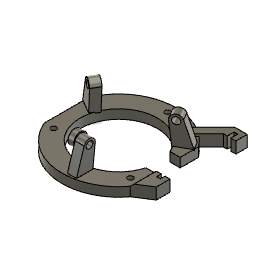
aball_v15 (Autodesk Fusion 360 design; units mm, degrees)
Autodesk Fusion 360 part; units mm, degrees
(part 1 of 2)
sphere "SpherePrimitive1" add diameter 38.1 placed x (1, 0, 0) y (0, 0, -1) z (0, 1, 0) at (0, 0, 0) makes body 1
ref_plane "WorkPlane1" through (0, -19.05, 0) normal (0, 1, 0) x (0, 0, 1)
mesh "Mesh1" [no effect]
ref_plane "WorkPlane2" through (0, -17.55, 0) normal (0, 1, 0) x (0, 0, 1)
sketch "bearing_38" plane through (0, 0, 0) normal (1, 0, 0) x (0, 0, -1)
  circle A0 centre (0, 0) radius 22.05 construction
  circle A1 centre (-18.1301, -12.55) radius 3
  circle A2 centre (-18.1301, -12.55) radius 1.5
  line L0 (-30, 0) -> (28, 0) construction
  line L1 (-30, -19.05) -> (30, -19.05) construction
  dimension "d13" = 44.1
  dimension "d14" = 6
  dimension "d15" = 3
  dimension "d16" = 19.05
  dimension "d17" = 6.5
  constraint coincident A0.centre origin
  constraint coincident A0 A1.centre
  constraint concentric A1 A2
  constraint horizontal L0
  constraint horizontal L1
  measures "d13" diameter of A0
  measures "d14" diameter of A1
  measures "d15" diameter of A2
  measures "d16" distance of L0 L1
  measures "d17" distance of A1.centre L1
sketch "bearing_holder_38" plane through (0, 0, 0) normal (1, 0, 0) x (0, 0, -1)
  circle A0 centre (-18.1301, -12.55) radius 2.5
  line L0 (-24.0474, -23.0415) -> (-20.5151, -11.8006)
  line L1 (-15.6305, -12.5064) -> (-16.7406, -23.0415)
  line L2 (-16.7406, -23.0415) -> (-24.0474, -23.0415)
  line L3 (0, -14.55) -> (0, -11.55)
  circle A1 centre (-18.1301, -12.55) radius 1.5
  point P0 (0, -13.05)
  point P1 (-18.1301, -12.55)
  dimension "d18" = 5
  constraint coincident A0 L0.end
  constraint tangent A0 L0
  constraint coincident A0 L1.start
  constraint horizontal L2
  constraint coincident P1 A0.centre
  measures "d18" diameter of A0
extrude "Extrude1" add sketch "bearing_38" along normal mid plane 2.5 separate body makes body 2
sketch "a9800_dimensino" plane through (0, 0, 0) normal (0, 1, 0) x (1, 0, 0)
  circle A0 centre (0, 0) radius 15.8
  line L0 (9.75, -10.75) -> (-9.75, -10.75)
  line L1 (-9.75, -10.75) -> (-9.75, 10.75)
  line L2 (-9.75, 10.75) -> (9.75, 10.75)
  line L3 (9.75, 10.75) -> (9.75, -10.75)
  line L4 (9.75, -10.75) -> (-9.75, 10.75) construction
  line L5 (-9.75, -10.75) -> (9.75, 10.75) construction
  line L6 (7.5, -8) -> (-7.5, -8)
  line L7 (-7.5, -8) -> (-7.5, 8)
  line L8 (-7.5, 8) -> (7.5, 8)
  line L9 (7.5, 8) -> (7.5, -8)
  line L10 (7.5, -8) -> (-7.5, 8) construction
  line L11 (-7.5, -8) -> (7.5, 8) construction
  circle A1 centre (0, 13.05) radius 1.25
  line L12 (-1.5901, 14.3) -> (1.6928, 14.3) construction
  line L13 (-2.2181, 15.8) -> (-2, 15.8)
  line L14 (-2, 15.8) -> (2, 15.8) construction
  circle A2 centre (0, -13.05) radius 1.25
  line L15 (-3.1209, -14.3) -> (2.5, -14.3) construction
  line L16 (-3, -15.8) -> (2.5, -15.8) construction
  line L17 (0, 40) -> (0, -43.8332) construction
  dimension "d32" = 31.6
  dimension "d33" = 21.5
  dimension "d34" = 19.5
  dimension "d35" = 15
  dimension "d36" = 16
  dimension "d37" = 2.5
  dimension "d38" = 1.5
  dimension "d39" = 2.5
  dimension "d40" = 1.5
  constraint coincident A0.centre origin
  constraint perpendicular L0 L1
  constraint parallel L0 L2
  constraint parallel L1 L3
  constraint horizontal L0
  constraint coincident L4 A0.centre
  constraint coincident L5 A0.centre
  constraint perpendicular L6 L7
  constraint parallel L6 L8
  constraint parallel L7 L9
  constraint horizontal L6
  constraint coincident L10 A0.centre
  constraint coincident L11 A0.centre
  constraint horizontal L12
  constraint parallel L12 L13
  constraint parallel L12 L14
  constraint tangent A0 L14
  constraint tangent A1 L12
  constraint horizontal L15
  constraint horizontal L16
  constraint tangent A0 L16
  constraint vertical L17
  constraint coincident A2.centre L17
  constraint tangent A2 L15
  measures "d32" diameter of A0
  measures "d33" distance of L0.end L1.end
  measures "d34" distance of L1.end L2.end
  measures "d35" distance of L7.end L8.end
  measures "d36" distance of L6.end L7.end
  measures "d37" diameter of A1
  measures "d38" distance of L12 L14
  measures "d39" diameter of A2
  measures "d40" distance of L15 L16
extrude "Extrude4" add sketch "a9800_dimensino" along normal blind 1.7 separate body contours A0 | L0 L1 L2 L3 | L6 L7 L8 L9 makes body 3
extrude "Extrude5" add sketch "a9800_dimensino" along normal blind 5 separate body contours L0 L1 L2 L3 | L6 L7 L8 L9 makes body 4
extrude "Extrude6" add sketch "a9800_dimensino" against normal blind 3 separate body contours L6 L7 L8 L9 makes body 5
combine "Combine3" operation add target body 3 tool bodies 4 5
copy_body "CopyPasteBodies3" bodies 3 makes body 6
move_body "Move4" bodies 6 to x (1, 0, 0) y (0, 1, 0) z (0, 0, 1) at (0, -30, 0)
move_body "Move5" bodies 6 to x (1, 0, 0) y (0, 1, 0) z (0, 0, 1) at (0, 3, 0)
move_body "Move6" bodies 6 to x (1, 0, 0) y (0, 1, 0) z (0, 0, 1) at (0, 2, 0)
move_body "Move7" bodies 6 to x (1, 0, 0) y (0, 1, 0) z (0, 0, 1) at (0, 0.15, 0)
move_body "Move8" bodies 6 to x (1, 0, 0) y (0, 1, 0) z (0, 0, 1) at (0, 0.5, 0)
move_face "MoveFace1" by (0, 0.02, 0) 1 faces at (-9.75, -20.45, 3.5833) on bodies 6
move_body "Move9" bodies 6 to x (1, 0, 0) y (0, 1, 0) z (0, 0, 1) at (0, 0.2, 0)
move_body "Move10" bodies 6 to x (1, 0, 0) y (0, 1, 0) z (0, 0, 1) at (0, -2.3, 0)
move_body "Move11" bodies 6 to x (1, 0, 0) y (0, 1, 0) z (0, 0, 1) at (0, 0.1, 0)
move_body "Move12" bodies 6 to x (0.34202, 0.939693, 0) y (-0.939693, 0.34202, 0) z (0, 0, 1) at (0, 0, 0)
ref_plane "WorkPlane5" through (0, -28, 0) normal (0, 1, 0) x (0, 0, 1)
ref_plane "WorkPlane6" through (0, -11, 0) normal (0, 1, 0) x (0, 0, 1)
ref_plane "WorkPlane7" through (0, -26.5, 0) normal (0, 1, 0) x (0, 0, 1)
move_body "Move13" bodies 6 to x (0, 0, -1) y (0, 1, 0) z (1, 0, 0) at (0, 0, 0)
mesh "Mesh2" [no effect]
sketch "Kyria_footprint" plane through (46, -28, 42) normal (0, 1, 0) x (1, 0, 0)
  line L0 (-210.8879, -20.4424) -> (-220.8051, -30.3595)
  circle A0 centre (-87.084, 9.634) radius 1.1
  arc A1 (-165.3859, -1.5948) -> (-210.8879, -20.4424) centre (-165.3859, -65.9444) ccw
  arc A2 (-128.8109, 1.9052) -> (-132.3109, -1.5948) centre (-132.3109, 1.9052) cw
  line L1 (-83.425, 74.1919) -> (-83.425, 9.475)
  arc A3 (-205.7208, 93.1275) -> (-85.2151, 77.2458) centre (-165.3859, -65.9444) cw
  circle A4 centre (-231.9682, 80.7528) radius 1.1
  circle A5 centre (-86.7356, 74.2991) radius 1.1
  circle A6 centre (-243.225, 19.2739) radius 1.1
  circle A7 centre (-256.3598, 5.4201) radius 1.1
  arc A8 (-85.2151, 77.2458) -> (-83.425, 74.1919) centre (-86.925, 74.1919) cw
  circle A9 centre (-223.2799, -27.6598) radius 1.1
  arc A10 (-245.225, 52.0721) -> (-246.225, 53.0721) centre (-245.225, 53.0721) cw
  arc A11 (-259.0595, 2.9452) -> (-259.0595, 7.8949) centre (-256.5847, 5.4201) cw
  line L2 (-228.225, 77.6065) -> (-207.475, 77.6065)
  arc A12 (-220.8051, -30.3595) -> (-225.7548, -30.3595) centre (-223.2799, -27.8847) cw
  arc A13 (-239.225, 51.0721) -> (-240.225, 52.0721) centre (-240.225, 51.0721) ccw
  line L3 (-225.7548, -30.3595) -> (-259.0595, 2.9452)
  line L4 (-240.225, 52.0721) -> (-245.225, 52.0721)
  arc A14 (-206.475, 92.1582) -> (-205.7208, 93.1275) centre (-205.475, 92.1582) cw
  arc A15 (-249.1424, 17.8121) -> (-239.5985, 26.3746) centre (-165.3859, -65.9444) cw
  line L5 (-246.225, 53.0721) -> (-246.225, 74.8141)
  arc A16 (-244.4104, 77.8815) -> (-230.6225, 84.6377) centre (-165.3859, -65.9444) cw
  arc A17 (-229.225, 78.6065) -> (-228.225, 77.6065) centre (-228.225, 78.6065) ccw
  arc A18 (-125.3109, 5.975) -> (-128.8109, 2.475) centre (-125.3109, 2.475) ccw
  arc A19 (-230.6225, 84.6377) -> (-229.225, 83.7201) centre (-230.225, 83.7201) cw
  arc A20 (-207.475, 77.6065) -> (-206.475, 78.6065) centre (-207.475, 78.6065) ccw
  line L6 (-259.0595, 7.8949) -> (-249.1424, 17.8121)
  arc A21 (-246.225, 74.8141) -> (-244.4104, 77.8815) centre (-242.725, 74.8141) cw
  line L7 (-229.225, 83.7201) -> (-229.225, 78.6065)
  line L8 (-128.8109, 2.475) -> (-128.8109, 1.9052)
  line L9 (-132.3109, -1.5948) -> (-165.3859, -1.5948)
  line L10 (-86.925, 5.975) -> (-125.3109, 5.975)
  arc A22 (-83.425, 9.475) -> (-86.925, 5.975) centre (-86.925, 9.475) cw
  arc A23 (-239.5985, 26.3746) -> (-239.225, 27.154) centre (-240.225, 27.154) ccw
  line L11 (-239.225, 27.154) -> (-239.225, 51.0721)
  line L12 (-206.475, 78.6065) -> (-206.475, 92.1582)
  circle A24 centre (-243.225, 55.0721) radius 1.1
  circle A25 centre (-203.5672, 90.5701) radius 1.1
copy_body "CopyPasteBodies6" bodies 2 makes body 7
move_body "Move16" bodies 7 to x (-0.5, 0, -0.866025) y (0, 1, 0) z (0.866025, 0, -0.5) at (0, 0, 0)
copy_body "CopyPasteBodies7" bodies 2 makes body 8
move_body "Move22" bodies 6 to x (1, 0, 0) y (0, 0.34202, -0.939693) z (0, 0.939693, 0.34202) at (0, 0, 0)
move_body "Move17" bodies 8 to x (-0.5, 0, 0.866025) y (0, 1, 0) z (-0.866025, 0, -0.5) at (0, 0, 0)
move_body "Move23" bodies 6 to x (0, 0, -1) y (0, 1, 0) z (1, 0, 0) at (0, 0, 0)
sketch "holder" plane through (0, -26.5, 0) normal (0, 1, 0) x (1, 0, 0)
  circle A0 centre (0, 0) radius 25
  circle A1 centre (0, 0) radius 17
  line L0 (0, 0) -> (25, 0) construction
  line L1 (0, 0) -> (25, 0) construction
  line L2 (20, 18) -> (20, -15)
  circle A2 centre (-18.8875, -9.75) radius 1.2
  circle A3 centre (0, 21.5) radius 1.2
  circle A4 centre (16.8875, -11.75) radius 1.2
  line L3 (-23, 13) -> (-23, -12)
  dimension "d162" = 50
  dimension "d163" = 34
  dimension "d242" = 2.4
  dimension "d243" = 2.4
  dimension "d244" = 2.4
  constraint coincident A0.centre A1.centre
  constraint concentric A0 A1
  constraint horizontal L0
  constraint horizontal L1
  constraint vertical L2
  constraint vertical L3
  measures "d162" diameter of A0
  measures "d163" diameter of A1
  measures "d242" diameter of A2
  measures "d243" diameter of A3
  measures "d244" diameter of A4
extrude "Extrude27" add sketch "holder" along normal blind 4 separate body contours A0 L2 L3 makes body 9
extrude "Extrude28" add sketch "bearing_holder_38" along normal blind 4 from surface at 1.25 separate body contours A0 L1 | A0 L0 L1 L2 picked at (-15.9906, -12.7979) makes body 10
pattern_circular "C-Pattern1" count 3 over 360 about axis through (0, 1.75, 0) along (0, 1, 0) of bodies 10 makes body 11 at (14.5414, -20.0098, -14.4576) makes body 12 at (-19.7914, -20.0098, -5.3644)
sketch "micro_holder" plane through (0, -26.5, 0) normal (0, 1, 0) x (1, 0, 0)
  line L0 (23.2, -6.5) -> (24.8, -6.5)
  line L1 (20, -10.5) -> (20, -6.5)
  line L2 (23.2, -6.5) -> (23.2, -4.5)
  line L3 (23.2, -4.5) -> (20, -4.5)
  line L4 (20, -4.5) -> (20, -6.5)
  line L5 (24.8, -4.5) -> (27, -4.5)
  line L6 (24.8, -6.5) -> (24.8, -4.5)
  line L7 (24.8, 27.5) -> (23.2, 27.5)
  line L8 (21.5, 27.5) -> (21.5, 29.5)
  line L9 (21.5, 29.5) -> (27, 29.5)
  line L10 (27, 24.5) -> (24.8, 24.5)
  line L11 (24.8, 24.5) -> (24.8, 27.5)
  line L12 (23.2, 27.5) -> (23.2, 24.5)
  line L13 (23.2, 24.5) -> (21.5, 24.5)
  line L14 (21.5, 24.5) -> (21.5, 27.5)
  line L15 (21.5, 29.5) -> (9.7205, 17.7205)
  line L16 (21.5, 29.5) -> (34.4035, 29.5) construction
  line L17 (21.5, 24.5) -> (12.8239, 15.8239)
  line L18 (21.5, 24.5) -> (30.0147, 24.5) construction
  line L19 (9.7205, 17.7205) -> (12.8239, 15.8239)
  line L20 (27, -10.5) -> (20, -15)
  line L21 (20, -15) -> (20, -10.5)
  line L22 (27, 24.5) -> (27, 29.5)
  line L23 (27, -4.5) -> (27, -10.5)
  dimension "d200" = 4
  dimension "d201" = 135
  dimension "d202" = 135
  dimension "d383" = 1.6
  constraint horizontal L0
  constraint vertical L1
  constraint vertical L2
  constraint horizontal L3
  constraint vertical L4
  constraint horizontal L5
  constraint vertical L6
  constraint horizontal L7
  constraint vertical L8
  constraint horizontal L9
  constraint horizontal L10
  constraint vertical L11
  constraint vertical L12
  constraint horizontal L13
  constraint vertical L14
  constraint coincident L7 L8.start
  constraint horizontal L16
  constraint horizontal L18
  constraint collinear L6 L11
  constraint perpendicular L16 L22
  constraint collinear L2 L12
  measures "d200" distance of L1.end L1.start
  measures "d201" angle of L15 L16
  measures "d202" angle of L17 L18
  measures "d383" distance of L2 L5.start
sketch "case_body_guides" plane through (0, -28, 0) normal (0, 1, 0) x (1, 0, 0)
  line L0 (0, 70) -> (0, -60) construction
  line L1 (34, 26.9443) -> (34, -18.401)
  line L2 (11.4009, -41) -> (-25, -41)
  line L3 (-29, -37) -> (-29, 26.9855)
  arc A0 (30.9987, 30.8176) -> (-25.993, 30.8603) centre (2.4198, -80.0119) ccw
  arc A1 (-25.993, 30.8603) -> (-29, 26.9855) centre (-25, 26.9855) ccw
  arc A2 (-29, -37) -> (-25, -41) centre (-25, -37) ccw
  arc A3 (34, 26.9443) -> (30.9987, 30.8176) centre (30, 26.9443) ccw
  line L4 (-23, -31) -> (-23, 22.3021)
  arc A4 (28.16, 25.4237) -> (-19.8196, 26.2173) centre (2.4198, -80.0119) ccw
  line L5 (18.1274, 27.3776) -> (21.5156, 31.1472)
  line L6 (29.1545, 31.2768) -> (29.1545, 28.4999)
  line L7 (29.1545, 28.4999) -> (28.1728, 28.4999)
  line L8 (28.16, 25.4237) -> (28.1728, 28.4999)
  line L9 (32.8284, -21.2294) -> (14.2294, -39.8284)
  line L10 (26.8132, -18.7593) -> (11.7441, -33.8284)
  arc A5 (11.4009, -41) -> (14.2294, -39.8284) centre (11.4009, -37) ccw
  arc A6 (32.8284, -21.2294) -> (34, -18.401) centre (30, -18.401) ccw
  line L11 (-19, -35) -> (8.9157, -35)
  line L12 (27.9847, -15.9479) -> (28.16, 25.4237)
  circle A7 centre (-25, -37) radius 1.2
  arc A8 (-23, -31) -> (-19, -35) centre (-19, -31) ccw
  arc A9 (8.9157, -35) -> (11.7441, -33.8284) centre (8.9157, -31) ccw
  arc A10 (26.8132, -18.7593) -> (27.9847, -15.9479) centre (23.9848, -15.9309) ccw
  arc A11 (-19.8196, 26.2173) -> (-23, 22.3021) centre (-19, 22.3021) ccw
  circle A12 centre (-25, -37) radius 1.75
  circle A13 centre (-25, 26.9855) radius 1.2
  circle A14 centre (-25, 26.9855) radius 1.75
  circle A15 centre (17, 31) radius 1.2
  circle A16 centre (17, 31) radius 1.75
  circle A17 centre (31, 26) radius 1.2
  circle A18 centre (31, 26) radius 1.75
  circle A19 centre (11, -38) radius 1.2
  circle A20 centre (11, -38) radius 1.75
  circle A21 centre (31, -18) radius 1.2
  circle A22 centre (31, -18) radius 1.75
  line L13 (21.5156, 31.1472) -> (21.5156, 32.8388)
  circle A23 centre (31, 4) radius 1.2
  circle A24 centre (31, 4) radius 1.75
  line L14 (28.0545, 0.5306) -> (34, 0.5306)
  line L15 (28.0414, -2.5651) -> (34, -2.5651)
  point P0 (34, 30)
  point P1 (34, -41)
  dimension "d213" = 71
  dimension "d214" = 4
  dimension "d217" = 6
  dimension "d218" = 4
  dimension "d219" = 4
  dimension "d220" = 2.4
  dimension "d221" = 4
  dimension "d222" = 3.5
  dimension "d223" = 2.4
  dimension "d224" = 3.5
  dimension "d225" = 2.4
  dimension "d226" = 3.5
  dimension "d227" = 2.4
  dimension "d228" = 3.5
  dimension "d229" = 2.4
  dimension "d230" = 3.5
  dimension "d231" = 2.4
  dimension "d232" = 3.5
  dimension "d320" = 2.4
  dimension "d321" = 3.5
  constraint vertical L0
  constraint vertical L1
  constraint horizontal L2
  constraint vertical L3
  constraint tangent A0 A1
  constraint tangent L3 A1
  constraint tangent L3 A2
  constraint tangent L2 A2
  constraint equal A1 A2
  constraint coincident P1 L2
  constraint coincident P1 L1
  constraint coincident P0 L1
  constraint coincident P0 A0
  constraint tangent L1 A3
  constraint tangent A0 A3
  constraint equal A1 A3
  constraint coincident A4 L5.start
  constraint coincident A0 L6.start
  constraint perpendicular L6 L7
  constraint parallel L9 L10
  constraint parallel L3 L4
  constraint concentric A0 A4
  constraint tangent L9 A5
  constraint tangent L2 A5
  constraint tangent L1 A6
  constraint tangent L9 A6
  constraint concentric A2 A7
  constraint tangent L4 A8
  constraint tangent L11 A8
  constraint tangent L11 A9
  constraint tangent L10 A9
  constraint equal A8 A9
  constraint tangent L10 A10
  constraint tangent L12 A10
  constraint equal A8 A10
  constraint tangent A4 A11
  constraint tangent L4 A11
  constraint equal A8 A11
  constraint concentric A7 A12
  constraint concentric A1 A13
  constraint concentric A1 A14
  constraint concentric A15 A16
  constraint concentric A17 A18
  constraint concentric A19 A20
  constraint concentric A21 A22
  constraint coincident A0 L13.end
  constraint vertical L13
  constraint concentric A23 A24
  constraint coincident L12 L14.start
  constraint coincident L1 L14.end
  constraint perpendicular L1 L14
  constraint coincident L12 L15.start
  constraint coincident L1 L15.end
  constraint perpendicular L1 L15
  measures "d213" distance of P0 P1
  measures "d214" radius of A1
  measures "d217" distance of L9 L10
  measures "d218" radius of A5
  measures "d219" radius of A6
  measures "d220" diameter of A7
  measures "d221" radius of A8
  measures "d222" diameter of A12
  measures "d223" diameter of A13
  measures "d224" diameter of A14
  measures "d225" diameter of A15
  measures "d226" diameter of A16
  measures "d227" diameter of A17
  measures "d228" diameter of A18
  measures "d229" diameter of A19
  measures "d230" diameter of A20
  measures "d231" diameter of A21
  measures "d232" diameter of A22
  measures "d320" diameter of A23
  measures "d321" diameter of A24
sketch "BOTTOM" plane through (0, -28, 0) normal (0, 1, 0) x (1, 0, 0)
  arc A0 (30.9987, 30.8176) -> (-25.993, 30.8603) centre (2.4198, -80.0119) ccw
  arc A1 (-25.993, 30.8603) -> (-29, 26.9855) centre (-25, 26.9855) ccw
  line L0 (-29, -37) -> (-29, 26.9855)
  arc A2 (34, 26.9443) -> (30.9987, 30.8176) centre (30, 26.9443) ccw
  line L1 (34, 26.9443) -> (34, -18.401)
  arc A3 (32.8284, -21.2294) -> (34, -18.401) centre (30, -18.401) ccw
  line L2 (32.8284, -21.2294) -> (14.2294, -39.8284)
  arc A4 (11.4009, -41) -> (14.2294, -39.8284) centre (11.4009, -37) ccw
  line L3 (11.4009, -41) -> (-25, -41)
  arc A5 (-29, -37) -> (-25, -41) centre (-25, -37) ccw
  circle A6 centre (-25, -37) radius 1.2
  circle A7 centre (11, -38) radius 1.2
  circle A8 centre (31, -18) radius 1.2
  circle A9 centre (31, 26) radius 1.2
  circle A10 centre (17, 31) radius 1.2
  circle A11 centre (-25, 26.9855) radius 1.2
  circle A12 centre (-18.8875, -9.75) radius 1.2
  circle A13 centre (16.8875, -11.75) radius 1.2
  circle A14 centre (0, 21.5) radius 1.2
  circle A15 centre (0, 13.0504) radius 1.2
  circle A16 centre (0, -13.05) radius 1.2
  arc A17 (-6.9032, 13.9049) -> (6.9032, 13.9049) centre (0, 18.0543) ccw
  arc A18 (6.9032, -13.9049) -> (-6.9032, -13.9049) centre (0, -18.0543) ccw
  arc A19 (-6.9032, 13.9049) -> (-6.9032, -13.9049) centre (0, 0) ccw
  arc A20 (6.9032, -13.9049) -> (6.9032, 13.9049) centre (0, 0) ccw
  circle A21 centre (31, 4) radius 1.2
  point P0 (-18.8875, -9.75)
  point P1 (34, 0.5306)
  dimension "d258" = 2.4
  dimension "d259" = 2.4
  constraint coincident A19.centre A20.centre
  constraint coincident A18.start A19
  constraint concentric A19 A20
  measures "d258" diameter of A15
  measures "d259" diameter of A16
extrude "Extrude29" add sketch "micro_holder" along normal blind 5 separate body makes body 13 at (17.5735, -24.8333, -25.5735) makes body 14 at (23.4, -26.5, 10.6667)
combine "Combine8" operation add target body 9 tool bodies 13 10 12 11 14
chamfer "Chamfer3" distance 1 angle 45 1 edges at (20, -21.5, 9.75) on bodies 9
chamfer "Chamfer4" distance 1 angle 45 1 edges at (11.2722, -21.5, -16.7722) on bodies 9
extrude "Extrude30" add sketch "BOTTOM" along normal blind 1.5 separate body makes body 15
extrude "Extrude31" add sketch "Kyria_footprint" along normal blind 17 separate body makes body 16
sketch "MIDDLEA" plane through (0, -26.5, 0) normal (0, 1, 0) x (1, 0, 0)
  line L0 (-29, -37) -> (-29, 26.9855)
  arc A0 (-25.993, 30.8603) -> (-29, 26.9855) centre (-25, 26.9855) ccw
  circle A1 centre (-25, 26.9855) radius 1.75
  arc A2 (-19.8196, 26.2173) -> (-23, 22.3021) centre (-19, 22.3021) ccw
  arc A3 (18.1274, 27.3776) -> (-19.8196, 26.2173) centre (2.4198, -80.0119) ccw
  line L1 (-23, -31) -> (-23, 22.3021)
  line L2 (18.1274, 27.3776) -> (21.5156, 31.1472)
  line L3 (29.1545, 31.2768) -> (29.1545, 28.4999)
  line L4 (29.1545, 28.4999) -> (28.1728, 28.4999)
  line L5 (28.16, 25.4237) -> (28.1728, 28.4999)
  circle A4 centre (31, 26) radius 1.75
  arc A5 (34, 26.9443) -> (30.9987, 30.8176) centre (30, 26.9443) ccw
  line L6 (27.9847, -15.9479) -> (28.16, 25.4237)
  line L7 (34, 26.9443) -> (34, -18.401)
  arc A6 (32.8284, -21.2294) -> (34, -18.401) centre (30, -18.401) ccw
  arc A7 (26.8132, -18.7593) -> (27.9847, -15.9479) centre (23.9848, -15.9309) ccw
  circle A8 centre (31, -18) radius 1.75
  line L8 (32.8284, -21.2294) -> (14.2294, -39.8284)
  line L9 (26.8132, -18.7593) -> (11.7441, -33.8284)
  arc A9 (11.4009, -41) -> (14.2294, -39.8284) centre (11.4009, -37) ccw
  arc A10 (8.9157, -35) -> (11.7441, -33.8284) centre (8.9157, -31) ccw
  circle A11 centre (11, -38) radius 1.75
  line L10 (11.4009, -41) -> (-25, -41)
  line L11 (-19, -35) -> (8.9157, -35)
  arc A12 (-23, -31) -> (-19, -35) centre (-19, -31) ccw
  arc A13 (-29, -37) -> (-25, -41) centre (-25, -37) ccw
  circle A14 centre (-25, -37) radius 1.75
  circle A15 centre (17, 31) radius 1.75
  line L12 (21.5156, 31.1472) -> (21.5156, 32.8388)
  arc A16 (30.9987, 30.8176) -> (29.1545, 31.2768) centre (2.4198, -80.0119) ccw
  arc A17 (21.5156, 32.8388) -> (-25.993, 30.8603) centre (2.4198, -80.0119) ccw
  circle A18 centre (31, 4) radius 1.75
  constraint concentric A16 A17
ref_plane "WorkPlane10" through (0, -11.5, 0) normal (0, 1, 0) x (0, 0, 1)
sketch "topA" plane through (0, -11.5, 0) normal (0, 1, 0) x (-1, 0, 0)
  circle A0 centre (-31, -26) radius 1.75
  circle A1 centre (25, 37) radius 1.75
  circle A2 centre (-17, -31) radius 1.75
  circle A3 centre (-31, 18) radius 1.75
  circle A4 centre (-11, 38) radius 1.75
  circle A5 centre (25, -26.9855) radius 1.75
  line L0 (-18.1274, -27.3776) -> (-21.5156, -31.1472)
  line L1 (-21.5156, -31.1472) -> (-23.0477, -31.1472)
  line L2 (-23.0477, -31.1472) -> (-23.0477, -32.5688)
  arc A6 (-23.0477, -32.5688) -> (25.993, -30.8603) centre (-2.4198, 80.0119) ccw
  arc A7 (25.993, -30.8603) -> (29, -26.9855) centre (25, -26.9855) ccw
  line L3 (29, -26.9855) -> (29, 37)
  arc A8 (29, 37) -> (25, 41) centre (25, 37) ccw
  line L4 (25, 41) -> (-11.4009, 41)
  arc A9 (-11.4009, 41) -> (-14.2294, 39.8284) centre (-11.4009, 37) ccw
  line L5 (-14.2294, 39.8284) -> (-32.8284, 21.2294)
  arc A10 (-32.8284, 21.2294) -> (-34, 18.401) centre (-30, 18.401) ccw
  line L6 (-34, 18.401) -> (-34, -26.9443)
  arc A11 (-34, -26.9443) -> (-30.9987, -30.8176) centre (-30, -26.9443) ccw
  arc A12 (-30.9987, -30.8176) -> (-29.1545, -31.2768) centre (-2.4198, 80.0119) ccw
  line L7 (-29.1545, -31.2768) -> (-29.1545, -28.4999)
  line L8 (-29.1545, -28.4999) -> (-28.1728, -28.4999)
  line L9 (-28.1728, -28.4999) -> (-28.16, -25.4237)
  line L10 (-28.16, -25.4237) -> (-27.9847, 15.9479)
  arc A13 (-26.8132, 18.7593) -> (-27.9847, 15.9479) centre (-23.9848, 15.9309) ccw
  line L11 (-26.8132, 18.7593) -> (-11.7441, 33.8284)
  arc A14 (-8.9157, 35) -> (-11.7441, 33.8284) centre (-8.9157, 31) ccw
  line L12 (-8.9157, 35) -> (19, 35)
  arc A15 (23, 31) -> (19, 35) centre (19, 31) ccw
  line L13 (23, 31) -> (23, -22.3021)
  arc A16 (19.8196, -26.2173) -> (23, -22.3021) centre (19, -22.3021) ccw
  arc A17 (-18.1274, -27.3776) -> (19.8196, -26.2173) centre (-2.4198, 80.0119) ccw
  line L14 (29, 37) -> (29, -26.9855)
  arc A18 (25.993, -30.8603) -> (29, -26.9855) centre (25, -26.9855) ccw
  arc A19 (-30.9987, -30.8176) -> (25.993, -30.8603) centre (-2.4198, 80.0119) ccw
  line L15 (-11.4009, 41) -> (25, 41)
  arc A20 (29, 37) -> (25, 41) centre (25, 37) ccw
  arc A21 (-11.4009, 41) -> (-14.2294, 39.8284) centre (-11.4009, 37) ccw
  line L16 (-32.8284, 21.2294) -> (-14.2294, 39.8284)
  arc A22 (-32.8284, 21.2294) -> (-34, 18.401) centre (-30, 18.401) ccw
  line L17 (-34, -26.9443) -> (-34, 18.401)
  circle A23 centre (-31, 18) radius 1.2
  circle A24 centre (-11, 38) radius 1.2
  arc A25 (-34, -26.9443) -> (-30.9987, -30.8176) centre (-30, -26.9443) ccw
  circle A26 centre (-31, -26) radius 1.2
  circle A27 centre (-17, -31) radius 1.2
  circle A28 centre (25, -26.9855) radius 1.2
  circle A29 centre (25, 37) radius 1.2
  line L18 (-22.5, -28) -> (-25, -28)
  line L19 (-25, -28) -> (-25, 7)
  line L20 (-25, 7) -> (-22.5, 7)
  line L21 (-22.5, 7) -> (-22.5, -28)
  circle A30 centre (0, 0) radius 23
  circle A31 centre (0, 0) radius 17.5
  line L22 (0, 0) -> (21.5407, 0) construction
  line L23 (0, 0) -> (21.5407, 0) construction
  line L24 (0, 0) -> (21.5407, 0) construction
  line L25 (0, 0) -> (21.5407, 0) construction
  line L26 (0, 0) -> (21.5407, 0) construction
  line L27 (0, 0) -> (21.5407, 0) construction
  circle A32 centre (-2.4311, 13.7873) radius 9.5
  circle A33 centre (-10.7246, -8.999) radius 9.5
  circle A34 centre (13.1557, -4.7883) radius 9.5
  line L28 (-23.0477, -31.1472) -> (-22.5, -28)
  line L29 (-25, -28) -> (-29.1, -28)
  line L30 (-29.1, -28) -> (-29.1545, -28.4999)
  line L31 (-21.5156, -31.1472) -> (-21.5156, -32.8388)
  point P0 (-31, 18)
  dimension "d268" = 35
  dimension "d300" = 46
  dimension "d301" = 19
  dimension "d302" = 19
  dimension "d303" = 19
  constraint horizontal L18
  constraint vertical L19
  constraint horizontal L20
  constraint vertical L21
  constraint coincident A30.centre A31.centre
  constraint concentric A30 A31
  constraint horizontal L22
  constraint horizontal L23
  constraint horizontal L24
  constraint horizontal L25
  constraint horizontal L26
  constraint horizontal L27
  constraint vertical L31
  constraint coincident A6 L31.end
  measures "d268" diameter of A31
  measures "d300" diameter of A30
  measures "d301" diameter of A32
  measures "d302" diameter of A33
  measures "d303" diameter of A34
ref_plane "WorkPlane11" through (0, -10, 0) normal (0, 1, 0) x (0, 0, 1)
ref_plane "WorkPlane12" through (0, -8.5, 0) normal (0, 1, 0) x (0, 0, 1)
sketch "topC" plane through (0, -8.5, 0) normal (0, 1, 0) x (1, 0, 0)
  circle A0 centre (0, 0) radius 19
  line L0 (22.9701, 27.7101) -> (24.4724, 27.7101)
  line L1 (24.4724, 27.7101) -> (24.4724, -6.6306)
  line L2 (24.4724, -6.6306) -> (22.9701, -6.6306)
  line L3 (22.9701, -6.6306) -> (22.9701, 27.7101)
  line L4 (12.6019, -21.7825) -> (26.0559, -25.2289)
  line L5 (34.0004, 26.9508) -> (34, -18.401)
  arc A1 (34.0004, 26.9508) -> (30.9492, 30.8241) centre (29.9824, 26.924) ccw
  circle A2 centre (31, 26) radius 1.2
  circle A3 centre (31, -18) radius 1.2
  arc A4 (32.8284, -21.2294) -> (34, -18.401) centre (30, -18.401) ccw
  line L6 (1.4117, 24.935) -> (13.6846, 32.4672)
  arc A5 (26.0559, -25.2289) -> (29.8, -24.2573) centre (27.0485, -21.354) ccw
  arc A6 (30.9492, 30.8241) -> (17.6483, 33.4338) centre (2.2985, -80.0016) ccw
  line L7 (32.8284, -21.2294) -> (29.8, -24.2573)
  circle A7 centre (31, 4) radius 1.2
  arc A8 (17.6483, 33.4338) -> (13.6846, 32.4672) centre (16.899, 27.8963) ccw
  circle A9 centre (17, 31) radius 1.2
  arc A10 (12.6019, -21.7825) -> (9.654, -21.9727) centre (11.4197, -26.3977) ccw
  arc A11 (-1.0236, 23.9782) -> (1.4117, 24.935) centre (-2.4946, 31.2999) ccw
  arc A12 (-1.0236, 23.9782) -> (9.654, -21.9727) centre (0, 0) ccw
  dimension "d296" = 4
  dimension "d316" = 38
  dimension "d343" = 48
  constraint coincident A0.centre A12.centre
  constraint horizontal L0
  constraint vertical L1
  constraint horizontal L2
  constraint vertical L3
  constraint tangent L4 A5
  constraint tangent A6 A8
  constraint tangent L4 A10
  constraint coincident A1.end A6.start
  constraint coincident L5.start A1.start
  constraint coincident L5.end A4.end
  constraint tangent L6 A11
  constraint coincident A4.start L7.start
  measures "d296" radius of A5
  measures "d316" diameter of A0
  measures "d343" diameter of A12
sketch "TOPA_dxf" plane through (0, 0, 0) normal (0, 1, 0) x (1, 0, 0)
  arc A0 (-25.993, 30.8603) -> (-29, 26.9855) centre (-25, 26.9855) ccw
  line L0 (-29, -37) -> (-29, 26.9855)
  circle A1 centre (-25, 26.9855) radius 1.2
  circle A2 centre (17, 31) radius 1.2
  arc A3 (34, 26.9443) -> (30.9987, 30.8176) centre (30, 26.9443) ccw
  circle A4 centre (31, 26) radius 1.2
  line L1 (34, -18.401) -> (34, 26.9443)
  arc A5 (32.8284, -21.2294) -> (34, -18.401) centre (30, -18.401) ccw
  line L2 (32.8284, -21.2294) -> (14.2294, -39.8284)
  circle A6 centre (31, -18) radius 1.2
  circle A7 centre (11, -38) radius 1.2
  arc A8 (11.4009, -41) -> (14.2294, -39.8284) centre (11.4009, -37) ccw
  line L3 (-25, -41) -> (11.4009, -41)
  arc A9 (-29, -37) -> (-25, -41) centre (-25, -37) ccw
  circle A10 centre (-25, -37) radius 1.2
  line L4 (25, 20) -> (25, -7)
  line L5 (22.5, -7) -> (22.5, 28)
  line L6 (25, -7) -> (22.5, -7)
  arc A11 (5.1826, 16.715) -> (-10.5869, 13.9344) centre (0, 0) ccw
  arc A12 (-17.0669, -3.8692) -> (-6.7741, -16.1357) centre (0, 0) ccw
  arc A13 (11.8843, -12.8458) -> (17.361, 2.2013) centre (0, 0) ccw
  line L7 (25, 20) -> (28.1, 20)
  line L8 (29.1545, 31.2768) -> (29.1545, 28.4999)
  circle A14 centre (31, 4) radius 1.2
  arc A15 (30.9987, 30.8176) -> (29.1545, 31.2768) centre (2.4198, -80.0119) ccw
  arc A16 (21.5851, 32.827) -> (-25.993, 30.8603) centre (2.4198, -80.0119) ccw
  line L9 (28.1, 20) -> (28.1, 28.4958)
  line L10 (28.1, 28.4958) -> (29.1545, 28.4999)
  arc A17 (-22.631, 4.1035) -> (-17.0669, -3.8692) centre (-13.1557, 4.7883) ccw
  arc A18 (-10.5869, 13.9344) -> (-19.974, 11.4035) centre (-13.1557, 4.7883) ccw
  arc A19 (-19.974, 11.4035) -> (-22.631, 4.1035) centre (0, 0) ccw
  arc A20 (0.1113, -22.9997) -> (7.7618, -21.6507) centre (0, 0) ccw
  arc A21 (17.361, 2.2013) -> (19.8627, 11.5963) centre (10.7246, 8.999) ccw
  arc A22 (14.8692, 17.5473) -> (5.1826, 16.715) centre (10.7246, 8.999) ccw
  arc A23 (19.8627, 11.5963) -> (14.8692, 17.5473) centre (0, 0) ccw
  arc A24 (7.7618, -21.6507) -> (11.8843, -12.8458) centre (2.4311, -13.7873) ccw
  arc A25 (-6.7741, -16.1357) -> (0.1113, -22.9997) centre (2.4311, -13.7873) ccw
  line L11 (22.5, 28) -> (21.5851, 28)
  line L12 (21.5851, 28) -> (21.5851, 32.827)
  point P0 (31, 26)
  constraint coincident A11.start A12
  constraint concentric A11 A12
  constraint coincident A13.start A12
  constraint concentric A12 A13
  constraint concentric A15 A16
  constraint perpendicular L7 L9
  constraint coincident L8.end L10.end
  constraint concentric A17 A18
  constraint coincident A22.start A21
  constraint concentric A19 A20
  constraint concentric A21 A22
  constraint concentric A24 A25
  constraint coincident L5.end L11.start
  constraint perpendicular L5 L11
  constraint perpendicular L11 L12
sketch "topB" plane through (0, -10, 0) normal (0, 1, 0) x (1, 0, 0)
  line L0 (34, -18.401) -> (34, 26.9443)
  arc A0 (34, 26.9443) -> (30.9987, 30.8176) centre (30, 26.9443) ccw
  arc A1 (32.8284, -21.2294) -> (34, -18.401) centre (30, -18.401) ccw
  circle A2 centre (31, -18) radius 1.2
  circle A3 centre (31, 26) radius 1.2
  circle A4 centre (17, 31) radius 1.2
  line L1 (25, 28) -> (25, -7)
  line L2 (22.5, -7) -> (22.5, 28)
  line L3 (25, -7) -> (22.5, -7)
  arc A5 (21.5851, 32.827) -> (10.3322, 34.1692) centre (2.4198, -80.0119) ccw
  line L4 (32.8284, -21.2294) -> (21.3525, -32.7053)
  line L5 (0.9317, 29.537) -> (8.0583, 33.6444)
  line L6 (1.5613, -29.4728) -> (17.4888, -33.7406)
  arc A6 (10.3322, 34.1692) -> (8.0583, 33.6444) centre (10.0557, 30.1787) ccw
  arc A7 (-1.0413, 28.9813) -> (0.9317, 29.537) centre (-1.1507, 33.1502) ccw
  arc A8 (17.4888, -33.7406) -> (21.3525, -32.7053) centre (18.5241, -29.8769) ccw
  arc A9 (1.5613, -29.4728) -> (-1.8438, -28.9413) centre (-2.6161, -45.063) ccw
  arc A10 (-0.9707, 28.9837) -> (-1.8438, -28.9413) centre (0, 0) ccw
  arc A11 (5.1826, 16.715) -> (-10.5869, 13.9344) centre (0, 0) ccw
  arc A12 (-17.0669, -3.8692) -> (-6.7741, -16.1357) centre (0, 0) ccw
  arc A13 (11.8843, -12.8458) -> (17.361, 2.2013) centre (0, 0) ccw
  line L7 (25, 28) -> (29.2, 28)
  line L8 (29.2, 28) -> (29.2, 31.2659)
  arc A14 (30.9987, 30.8176) -> (29.2, 31.2659) centre (2.4198, -80.0119) ccw
  arc A15 (21.5851, 32.827) -> (10.3322, 34.1692) centre (2.4198, -80.0119) ccw
  circle A16 centre (31, 4) radius 1.2
  arc A17 (-19.974, 11.4035) -> (-22.631, 4.1035) centre (0, 0) ccw
  arc A18 (0.1113, -22.9997) -> (7.7618, -21.6507) centre (0, 0) ccw
  arc A19 (19.8627, 11.5963) -> (14.8692, 17.5473) centre (0, 0) ccw
  arc A20 (14.8692, 17.5473) -> (5.1826, 16.715) centre (10.7246, 8.999) ccw
  arc A21 (17.361, 2.2013) -> (19.8627, 11.5963) centre (10.7246, 8.999) ccw
  arc A22 (-22.631, 4.1035) -> (-17.0669, -3.8692) centre (-13.1557, 4.7883) ccw
  arc A23 (-10.5869, 13.9344) -> (-19.974, 11.4035) centre (-13.1557, 4.7883) ccw
  arc A24 (7.7618, -21.6507) -> (11.8843, -12.8458) centre (2.4311, -13.7873) ccw
  arc A25 (-6.7741, -16.1357) -> (0.1113, -22.9997) centre (2.4311, -13.7873) ccw
  line L9 (21.5851, 28) -> (21.5851, 32.827)
  line L10 (22.5, 28) -> (21.5851, 28)
  dimension "d306" = 58
  dimension "d309" = 4
  dimension "d310" = 4
  dimension "d311" = 35
  constraint concentric A10 A12
  constraint tangent L5 A6
  constraint tangent A5 A6
  constraint tangent L5 A7
  constraint coincident A7.start A10
  constraint tangent L6 A8
  constraint tangent L4 A8
  constraint tangent L6 A9
  constraint coincident A11.start A12
  constraint concentric A11 A12
  constraint concentric A12 A13
  constraint perpendicular L1 L7
  constraint perpendicular L7 L8
  constraint concentric A14 A15
  constraint coincident A7 A10.start
  constraint concentric A17 A18
  constraint concentric A18 A19
  constraint concentric A20 A21
  constraint concentric A22 A23
  constraint concentric A24 A25
  measures "d306" diameter of A10
  measures "d309" radius of A6
  measures "d310" radius of A8
  measures "d311" diameter of A12
extrude "Extrude40" add sketch "TOPA_dxf" along normal blind 2.9 separate body makes body 17
move_body "Move34" bodies 17 to x (1, 0, 0) y (0, 1, 0) z (0, 0, 1) at (0, -14.9, 0)
sketch "MIDDLEB" plane through (0, -28, 0) normal (0, 1, 0) x (1, 0, 0)
  arc A0 (21.5156, 32.8388) -> (-25.993, 30.8603) centre (2.4198, -80.0119) ccw
  arc A1 (18.1274, 27.3776) -> (-19.8196, 26.2173) centre (2.4198, -80.0119) ccw
  circle A2 centre (17, 31) radius 1.75
  line L0 (18.1274, 27.3776) -> (21.5156, 31.1472)
  line L1 (21.5156, 31.1472) -> (21.5156, 32.8388)
  line L2 (29.1545, 31.2768) -> (29.1545, 28.4999)
  arc A3 (30.9987, 30.8176) -> (29.1545, 31.2768) centre (2.4198, -80.0119) ccw
  arc A4 (34, 26.9443) -> (30.9987, 30.8176) centre (30, 26.9443) ccw
  line L3 (28.16, 25.4237) -> (28.1728, 28.4999)
  line L4 (29.1545, 28.4999) -> (28.1728, 28.4999)
  circle A5 centre (31, 26) radius 1.75
  circle A6 centre (31, 4) radius 1.75
  circle A7 centre (31, -18) radius 1.75
  arc A8 (32.8284, -21.2294) -> (34, -18.401) centre (30, -18.401) ccw
  arc A9 (26.8132, -18.7593) -> (27.9847, -15.9479) centre (23.9848, -15.9309) ccw
  line L5 (32.8284, -21.2294) -> (14.2294, -39.8284)
  line L6 (26.8132, -18.7593) -> (11.7441, -33.8284)
  line L7 (-19, -35) -> (8.9157, -35)
  arc A10 (8.9157, -35) -> (11.7441, -33.8284) centre (8.9157, -31) ccw
  arc A11 (11.4009, -41) -> (14.2294, -39.8284) centre (11.4009, -37) ccw
  line L8 (11.4009, -41) -> (-25, -41)
  circle A12 centre (11, -38) radius 1.75
  circle A13 centre (-25, -37) radius 1.75
  arc A14 (-23, -31) -> (-19, -35) centre (-19, -31) ccw
  arc A15 (-29, -37) -> (-25, -41) centre (-25, -37) ccw
  line L9 (-29, -37) -> (-29, 26.9855)
  line L10 (-23, -31) -> (-23, 22.3021)
  arc A16 (-19.8196, 26.2173) -> (-23, 22.3021) centre (-19, 22.3021) ccw
  circle A17 centre (-25, 26.9855) radius 1.75
  arc A18 (-25.993, 30.8603) -> (-29, 26.9855) centre (-25, 26.9855) ccw
  line L11 (28.0545, 0.5306) -> (34, 0.5306)
  line L12 (28.0414, -2.5651) -> (34, -2.5651)
  line L13 (27.9847, -15.9479) -> (28.0414, -2.5651)
  line L14 (28.0545, 0.5306) -> (28.16, 25.4237)
  line L15 (34, 26.9443) -> (34, 0.5306)
  line L16 (34, -2.5651) -> (34, -18.401)
  constraint collinear L13 L14
  constraint collinear L15 L16
extrude "Extrude41" add sketch "MIDDLEA" along normal blind 2.9 separate body makes body 18
extrude "Extrude42" add sketch "MIDDLEB" along normal blind 2.9 separate body makes body 19 at (-27, -28, 13.6715) makes body 20 at (29.47, -28, -18.4746)
move_body "Move35" bodies 19 20 to x (1, 0, 0) y (0, 1, 0) z (0, 0, 1) at (0, 4.4, 0)
copy_body "CopyPasteBodies20" bodies 19 20 makes body 21 makes body 22
move_body "Move36" bodies 21 22 to x (1, 0, 0) y (0, 1, 0) z (0, 0, 1) at (0, 2.9, 0)
copy_body "CopyPasteBodies21" bodies 18 makes body 23
move_body "Move37" bodies 23 to x (1, 0, 0) y (0, 1, 0) z (0, 0, 1) at (0, 8.7, 0)
copy_body "CopyPasteBodies22" bodies 17 makes body 24
move_body "Move38" bodies 24 to x (1, 0, 0) y (0, 1, 0) z (0, 0, 1) at (0, 5, 0)
move_body "Move39" bodies 24 to x (1, 0, 0) y (0, 1, 0) z (0, 0, 1) at (0, -5, 0)
combine "Combine9" operation add target body 24 tool bodies 22 21 20 19 23 18 keep tools
extrude "Extrude43" add sketch "topB" along normal blind 2.9 separate body makes body 25
move_body "Move40" bodies 25 to x (1, 0, 0) y (0, 1, 0) z (0, 0, 1) at (0, -2, 0)
move_body "Move42" bodies 16 to x (1, 0, 0) y (0, 1, 0) z (0, 0, 1) at (5, 1.5, 0)
move_body "Move43" bodies 16 to x (1, 0, 0) y (0, 1, 0) z (0, 0, 1) at (0, 0, 5)
extrude "Extrude45" add sketch "topC" along normal blind 2.9 separate body makes body 26
move_body "Move44" bodies 26 to x (1, 0, 0) y (0, 1, 0) z (0, 0, 1) at (0, -0.6, 0)
sketch "witre_channel" plane through (0, 0, 0) normal (0, 1, 0) x (1, 0, 0)
  line L0 (20.1, -4.5) -> (15, -4.5)
  line L1 (15, -4.5) -> (15, 7)
  line L2 (15, 7) -> (20.1, 7)
  line L3 (20.1, 7) -> (20.1, -4.5)
  dimension "d344" = 11.5
  constraint horizontal L0
  constraint vertical L1
  constraint horizontal L2
  constraint vertical L3
  measures "d344" distance of L0.start L2.end
extrude "Extrude46" cut sketch "witre_channel" against normal blind 30 bodies 9
ref_plane "WorkPlane13" through (0, -18.5, 0) normal (0, 1, 0) x (0, 0, 1)
sketch "plate_bottom" plane through (0, -26.5, 0) normal (0, 1, 0) x (1, 0, 0)
  line L0 (-22.9732, 30.9417) -> (27.0268, 30.9417)
  arc A0 (-22.9732, 30.9417) -> (-24.9732, 28.9417) centre (-22.9732, 28.9417) ccw
  line L1 (-24.9732, -26.5583) -> (-24.9732, 28.9417)
  arc A1 (-24.9732, -26.5583) -> (-22.9732, -28.5583) centre (-22.9732, -26.5583) ccw
  line L2 (12.4658, -28.5583) -> (-22.9732, -28.5583)
  arc A2 (12.4658, -28.5583) -> (13.8801, -27.9725) centre (12.4658, -26.5583) ccw
  line L3 (28.441, -13.4115) -> (13.8801, -27.9725)
  arc A3 (28.441, -13.4115) -> (29.0268, -11.9973) centre (27.0268, -11.9973) ccw
  line L4 (29.0268, 28.9417) -> (29.0268, -11.9973)
  arc A4 (29.0268, 28.9417) -> (27.0268, 30.9417) centre (27.0268, 28.9417) ccw
  arc A5 (-6.9032, 13.9049) -> (-6.9032, -13.9049) centre (0, 0) ccw
  arc A6 (-6.9032, 13.9049) -> (6.9032, 13.9049) centre (0, 18.0543) ccw
  arc A7 (6.9032, -13.9049) -> (6.9032, 13.9049) centre (0, 0) ccw
  arc A8 (6.9032, -13.9049) -> (-6.9032, -13.9049) centre (0, -18.0543) ccw
  circle A9 centre (16.8875, -11.75) radius 1.2
  circle A10 centre (0, -13.05) radius 1.2
  circle A11 centre (-18.8875, -9.75) radius 1.2
  circle A12 centre (0, 13.0504) radius 1.2
  circle A13 centre (0, 21.5) radius 1.2
  circle A14 centre (-22, -25) radius 1.2
  circle A15 centre (12.5, -25) radius 1.2
  circle A16 centre (-22, 28) radius 1.2
  circle A17 centre (15, 28) radius 1.2
  circle A18 centre (21.1605, -17.0818) radius 1.2
  dimension "d371" = 2.4
  dimension "d372" = 2.4
  dimension "d373" = 2.4
  dimension "d374" = 2.4
  dimension "d375" = 2.4
  measures "d371" diameter of A14
  measures "d372" diameter of A15
  measures "d373" diameter of A16
  measures "d374" diameter of A17
  measures "d375" diameter of A18
sketch "plate_mid" plane through (0, -18.5, 0) normal (0, 1, 0) x (1, 0, 0)
  line L0 (-24.9732, -26.5583) -> (-24.9732, 28.9417)
  arc A0 (-24.9732, -26.5583) -> (-22.9732, -28.5583) centre (-22.9732, -26.5583) ccw
  line L1 (12.4658, -28.5583) -> (-22.9732, -28.5583)
  arc A1 (12.4658, -28.5583) -> (13.8801, -27.9725) centre (12.4658, -26.5583) ccw
  line L2 (28.441, -13.4115) -> (13.8801, -27.9725)
  line L3 (29.0268, -10) -> (29.0268, -11.9973)
  arc A2 (28.441, -13.4115) -> (29.0268, -11.9973) centre (27.0268, -11.9973) ccw
  line L4 (-22.9732, 30.9417) -> (19.7938, 30.9417)
  arc A3 (-22.9732, 30.9417) -> (-24.9732, 28.9417) centre (-22.9732, 28.9417) ccw
  circle A4 centre (0, 0) radius 11
  line L5 (-21.8156, 10.6407) -> (-23.328, 8.1199)
  line L6 (-22.642, 5.376) -> (-17.5741, 2.3352)
  line L7 (-14.8301, 3.0212) -> (-13.3177, 5.5419)
  line L8 (-14.0037, 8.2859) -> (-19.0716, 11.3267)
  arc A5 (-19.0716, 11.3267) -> (-21.8156, 10.6407) centre (-20.1006, 9.6117) ccw
  arc A6 (-23.328, 8.1199) -> (-22.642, 5.376) centre (-21.613, 7.091) ccw
  arc A7 (-17.5741, 2.3352) -> (-14.8301, 3.0212) centre (-16.5451, 4.0502) ccw
  arc A8 (-13.3177, 5.5419) -> (-14.0037, 8.2859) centre (-15.0326, 6.5709) ccw
  line L9 (-0.174, -16.2705) -> (-0.2734, -22.1798)
  arc A9 (-0.2734, -22.1798) -> (1.6927, -24.2132) centre (1.7263, -22.2135) ccw
  line L10 (1.6927, -24.2132) -> (4.6319, -24.2626)
  arc A10 (4.6319, -24.2626) -> (6.6653, -22.2966) centre (4.6656, -22.2629) ccw
  line L11 (6.6653, -22.2966) -> (6.7647, -16.3872)
  arc A11 (6.7647, -16.3872) -> (4.7986, -14.3538) centre (4.765, -16.3536) ccw
  line L12 (4.7986, -14.3538) -> (1.8594, -14.3044)
  arc A12 (1.8594, -14.3044) -> (-0.174, -16.2705) centre (1.8257, -16.3041) ccw
  line L13 (14.1776, 7.9846) -> (19.345, 10.8531)
  arc A13 (19.345, 10.8531) -> (20.1229, 13.5725) centre (18.3743, 12.6018) ccw
  line L14 (20.1229, 13.5725) -> (18.6961, 16.1427)
  arc A14 (18.6961, 16.1427) -> (15.9767, 16.9206) centre (16.9475, 15.172) ccw
  line L15 (15.9767, 16.9206) -> (10.8094, 14.052)
  arc A15 (10.8094, 14.052) -> (10.0315, 11.3327) centre (11.7801, 12.3034) ccw
  line L16 (10.0315, 11.3327) -> (11.4583, 8.7625)
  arc A16 (11.4583, 8.7625) -> (14.1776, 7.9846) centre (13.2069, 9.7332) ccw
  line L17 (21.7938, 19.8987) -> (21.7938, 28.9417)
  line L18 (21.7938, 19.8987) -> (21.7938, -6)
  line L19 (23.7938, -8) -> (27.0268, -8)
  arc A17 (21.7938, 28.9417) -> (19.7938, 30.9417) centre (19.7938, 28.9417) ccw
  arc A18 (21.7938, -6) -> (23.7938, -8) centre (23.7938, -6) ccw
  arc A19 (29.0268, -10) -> (27.0268, -8) centre (27.0268, -10) ccw
  circle A20 centre (-22, 28) radius 1.2
  circle A21 centre (15, 28) radius 1.2
  circle A22 centre (12.5, -25) radius 1.2
  circle A23 centre (-22, -25) radius 1.2
  circle A24 centre (21.1605, -17.0818) radius 1.2
  dimension "d353" = 22
  dimension "d354" = 2
  dimension "d356" = 360
  dimension "d357" = 2
  constraint coincident A4.centre origin
  constraint perpendicular L5 L6
  constraint perpendicular L6 L7
  constraint perpendicular L7 L8
  constraint tangent L5 A5
  constraint tangent L8 A5
  constraint tangent L5 A6
  constraint tangent L6 A6
  constraint equal A5 A6
  constraint tangent L6 A7
  constraint tangent L7 A7
  constraint equal A5 A7
  constraint tangent L8 A8
  constraint tangent L7 A8
  constraint equal A5 A8
  constraint vertical L17
  constraint parallel L17 L18
  constraint perpendicular L3 L19
  constraint tangent L4 A17
  constraint tangent L17 A17
  constraint tangent L18 A18
  constraint tangent L19 A18
  constraint equal A17 A18
  constraint tangent L3 A19
  constraint tangent L19 A19
  constraint equal A17 A19
  measures "d353" diameter of A4
  measures "d354" radius of A5
  measures "d357" radius of A17
ref_plane "WorkPlane14" through (0, -8.5, 0) normal (0, 1, 0) x (0, 0, 1)
sketch "plate_top" plane through (0, -8.5, 0) normal (0, 1, 0) x (1, 0, 0)
  line L0 (12.8255, 30.9417) -> (27.0268, 30.9417)
  arc A0 (29.0268, 28.9417) -> (27.0268, 30.9417) centre (27.0268, 28.9417) ccw
  line L1 (29.0268, 28.9417) -> (29.0268, -11.9973)
  line L2 (28.441, -13.4115) -> (13.8801, -27.9725)
  arc A1 (28.441, -13.4115) -> (29.0268, -11.9973) centre (27.0268, -11.9973) ccw
  arc A2 (12.4658, -28.5583) -> (13.8801, -27.9725) centre (12.4658, -26.5583) ccw
  line L3 (12.4658, -28.5583) -> (10.4421, -28.5583)
  circle A3 centre (0, 0) radius 19
  line L4 (22.9701, 27.7101) -> (24.4724, 27.7101)
  line L5 (22.9701, -6.6306) -> (22.9701, 27.7101)
  line L6 (24.4724, 27.7101) -> (24.4724, -6.6306)
  line L7 (24.4724, -6.6306) -> (22.9701, -6.6306)
  line L8 (6.0554, 25) -> (11.4113, 30.3559)
  line L9 (6.5094, -25.454) -> (9.0279, -27.9725)
  arc A4 (12.8255, 30.9417) -> (11.4113, 30.3559) centre (12.8255, 28.9417) ccw
  arc A5 (9.0279, -27.9725) -> (10.4421, -28.5583) centre (10.4421, -26.5583) ccw
  arc A6 (4.6084, 24.5716) -> (6.5094, 25.454) centre (4.3533, 27.6101) ccw
  arc A7 (6.5094, -25.454) -> (4.3533, -24.6181) centre (4.4841, -27.4793) ccw
  arc A8 (4.6084, 24.5716) -> (4.3533, -24.6181) centre (0, 0) ccw
  circle A9 centre (12.5, -25) radius 1.2
  circle A10 centre (21.1605, -17.0818) radius 1.2
  circle A11 centre (15, 28) radius 1.2
  dimension "d363" = 38
  dimension "d364" = 50
  dimension "d368" = 2
  constraint coincident A3.centre A8.centre
  constraint tangent L8 A4
  constraint tangent L0 A4
  constraint tangent L9 A5
  constraint tangent L3 A5
  constraint equal A4 A5
  constraint tangent L8 A6
  constraint coincident L8 A6.end
  constraint tangent L9 A7
  measures "d363" diameter of A3
  measures "d364" diameter of A8
  measures "d368" radius of A4
extrude "Extrude50" add sketch "plate_bottom" against normal blind 1.5 separate body makes body 27
extrude "Extrude51" add sketch "plate_mid" along normal blind 1.5 separate body makes body 28
extrude "Extrude52" add sketch "plate_top" along normal blind 1.5 separate body makes body 29
sphere "SpherePrimitive2" add diameter 34 placed x (0, 0, -1) y (0, 1, 0) z (1, 0, 0) at (0, -20, -26) separate body makes body 30
move_body "MoveFace2" bodies 30 to x (1, 0, 0) y (0, 1, 0) z (0, 0, 1) at (0, 18, 26) on bodies 30
sketch "bearing_34" plane through (0, 0, 0) normal (1, 0, 0) x (0, 1, 0)
  line L0 (-30, -19.05) -> (30, -19.05)
  circle A0 centre (-13.1301, 16.65) radius 3
  line L1 (-30, 0) -> (28, 0)
  circle A1 centre (-13.1301, 16.65) radius 1.5
  circle A2 centre (-2, 0) radius 20 construction
  dimension "d386" = 40
  constraint coincident L1 A2.centre
  measures "d386" diameter of A2
sketch "bearing_holder_34" plane through (0, 0, 0) normal (1, 0, 0) x (0, 1, 0)
  line L0 (-23.015, 24.2097) -> (-12.0201, 19.0271)
  circle A0 centre (-13.15, 16.6301) radius 2.65
  circle A1 centre (-13.15, 16.6301) radius 1.5
  line L1 (-13.846, 14.0731) -> (-23.0269, 16.5721)
  line L2 (-23.0269, 16.5721) -> (-23.015, 24.2097)
  dimension "d399" = 5.3
  constraint coincident A0 L1.start
  constraint tangent A0 L1
  constraint coincident L0.end A0
  constraint tangent L0 A0
  measures "d399" diameter of A0
extrude "Extrude53" add sketch "holder" along normal blind 4 separate body contours A0 L2 L3 makes body 31
extrude "Extrude54" add sketch "micro_holder" along normal blind 5 bodies 31
chamfer "Chamfer5" distance 1 angle 45 1 edges at (20, -21.5, 9.75) on bodies 31
extrude "Extrude55" add sketch "bearing_holder_34" along normal blind 4 from surface at 1.25 separate body makes body 32
pattern_circular "C-Pattern2" count 3 over 360 about axis through (0, 1.75, 0) along (0, 1, 0) of bodies 32 makes body 33 at (16.1923, -20.1437, -10.792) makes body 34 at (-17.4423, -20.1437, -8.6269)
combine "Combine10" operation add target body 31 tool bodies 34 33 32
extrude "Extrude56" cut sketch "witre_channel" against normal blind 34 bodies 31
move_body "Move46" bodies 2 to x (1, 0, 0) y (0, 1, 0) z (0, 0, 1) at (0, -0.6, -1.5)
move_body "Move47" bodies 2 to x (1, 0, 0) y (0, 1, 0) z (0, 0, 1) at (0, 0.6, 1.5)
hidden bodies 1 3 6 7 8 16 24 27 28 29 30 31
equation "ball_size = 38.1 mm"
equation "bearing_dia_inside = 3 mm"
equation "bearing_dia_outside = 6 mm"
equation "Bearing_width = 2.5 mm"
equation "d5 = ball_size"
equation "d6 = -ball_size / 2"
equation "d7 = -( ball_size / 2 - 1.5 mm )"
equation "d13 = ball_size + bearing_dia_outside"
equation "d14 = bearing_dia_outside"
equation "d15 = bearing_dia_inside"
equation "d16 = ball_size / 2"
equation "d17 = bearingPlacement"
equation "d18 = bearing_dia_outside - 1 mm"
equation "d19 = Bearing_width"
equation "standoffDia = 3.5 mm"
equation "m2_screwhole = 2.4 mm"
equation "bearingPlacement = 6.5 mm"
equation "d220 = m2_screwhole"
equation "d222 = standoffDia"
equation "d223 = m2_screwhole"
equation "d224 = standoffDia"
equation "d225 = m2_screwhole"
equation "d226 = standoffDia"
equation "d227 = m2_screwhole"
equation "d228 = standoffDia"
equation "d229 = m2_screwhole"
equation "d230 = standoffDia"
equation "d231 = m2_screwhole"
equation "d232 = standoffDia"
equation "d242 = m2_screwhole"
equation "d243 = m2_screwhole"
equation "d244 = m2_screwhole"
equation "d248 = Bearing_width / 2"
equation "d258 = m2_screwhole"
equation "d259 = m2_screwhole"
equation "d320 = m2_screwhole"
equation "d321 = standoffDia"
equation "d371 = m2_screwhole"
equation "d372 = m2_screwhole"
equation "d373 = m2_screwhole"
equation "d374 = m2_screwhole"
equation "d375 = m2_screwhole"
equation "mcu_pcb_thickness = 1.6 mm"
equation "d383 = mcu_pcb_thickness"
equation "d386 = 34 mm + bearing_dia_outside"